Autodesk Fusion 360 part; units mm, degrees
note: some values were not read from the file. Set by a fixed rule: which sketch regions a step uses.
(part 9 of 20)
  spline S48 degree 5 poles (20.3781, 23.3609) (20.3757, 23.3596) (20.371, 23.3571) (20.3639, 23.3532) (20.3544, 23.348) (20.3426, 23.3416) (20.3308, 23.3351) (20.319, 23.3287) (20.3073, 23.3222) (20.2957, 23.3158) (20.284, 23.3094) (20.2724, 23.3029) (20.2609, 23.2965) (20.2493, 23.29) (20.2379, 23.2836) (20.2264, 23.2771) (20.215, 23.2707) (20.2036, 23.2643) (20.1922, 23.2578) (20.1809, 23.2514) (20.1697, 23.245) (20.1584, 23.2385) (20.1472, 23.2321) (20.136, 23.2257) (20.1249, 23.2193) (20.1138, 23.2128) (20.1028, 23.2064) (20.0917, 23.2) (20.0808, 23.1936) (20.0698, 23.1872) (20.0589, 23.1807) (20.048, 23.1743) (20.0372, 23.1679) (20.0264, 23.1615) (20.0156, 23.1551) (20.0049, 23.1487) (19.9942, 23.1423) (19.9836, 23.136) (19.973, 23.1296) (19.9624, 23.1232) (19.9518, 23.1168) (19.9413, 23.1104) (19.9309, 23.1041) (19.9205, 23.0977) (19.9101, 23.0914) (19.8997, 23.085) (19.8894, 23.0786) (19.8791, 23.0723) (19.8689, 23.066) (19.8587, 23.0596) (19.8486, 23.0533) (19.8384, 23.047) (19.8284, 23.0406) (19.8183, 23.0343) (19.8083, 23.028) (19.7984, 23.0217) (19.7884, 23.0154) (19.7785, 23.0091) (19.7687, 23.0029) (19.7589, 22.9966) (19.7491, 22.9903) (19.7394, 22.984) (19.7297, 22.9778) (19.72, 22.9715) (19.7104, 22.9653) (19.7009, 22.9591) (19.6913, 22.9528) (19.6818, 22.9466) (19.6724, 22.9404) (19.663, 22.9342) (19.6536, 22.928) (19.6443, 22.9218) (19.635, 22.9156) (19.6257, 22.9095) (19.6165, 22.9033) (19.6073, 22.8971) (19.5982, 22.891) (19.5891, 22.8849) (19.5801, 22.8787) (19.5711, 22.8726) (19.5621, 22.8665) (19.5532, 22.8604) (19.5443, 22.8543) (19.5354, 22.8483) (19.5266, 22.8422) (19.5179, 22.8361) (19.5091, 22.8301) (19.5005, 22.8241) (19.4918, 22.818) (19.4832, 22.812) (19.4747, 22.806) (19.4662, 22.8) (19.4577, 22.7941) (19.4493, 22.7881) (19.4409, 22.7822) (19.4325, 22.7762) (19.4242, 22.7703) (19.416, 22.7644) (19.4078, 22.7585) (19.3996, 22.7526) (19.3914, 22.7467) (19.3834, 22.7408) (19.3753, 22.735) (19.3673, 22.7292) (19.3593, 22.7233) (19.3514, 22.7175) (19.3436, 22.7118) (19.3357, 22.706) (19.3279, 22.7002) (19.3202, 22.6945) (19.3125, 22.6887) (19.3048, 22.683) (19.2972, 22.6773) (19.2897, 22.6716) (19.2821, 22.666) (19.2747, 22.6603) (19.2672, 22.6547) (19.2598, 22.6491) (19.2525, 22.6435) (19.2452, 22.6379) (19.2379, 22.6323) (19.2307, 22.6268) (19.2236, 22.6212) (19.2165, 22.6157) (19.2094, 22.6102) (19.2024, 22.6048) (19.1954, 22.5993) (19.1884, 22.5939) (19.1815, 22.5884) (19.1747, 22.583) (19.1679, 22.5777) (19.1611, 22.5723) (19.1544, 22.567) (19.1478, 22.5617) (19.1412, 22.5564) (19.1346, 22.5511) (19.1281, 22.5458) (19.1216, 22.5406) (19.1152, 22.5354) (19.1088, 22.5302) (19.1025, 22.525) (19.0962, 22.5199) (19.09, 22.5148) (19.0838, 22.5097) (19.0776, 22.5046) (19.0715, 22.4996) (19.0655, 22.4945) (19.0595, 22.4895) (19.0536, 22.4846) (19.0477, 22.4796) (19.0418, 22.4747) (19.036, 22.4698) (19.0303, 22.4649) (19.0246, 22.4601) (19.0189, 22.4553) (19.0133, 22.4505) (19.0077, 22.4457) (19.0022, 22.441) (18.9968, 22.4363) (18.9914, 22.4316) (18.986, 22.427) (18.9807, 22.4223) (18.9755, 22.4177) (18.9703, 22.4132) (18.9651, 22.4087) (18.96, 22.4042) (18.955, 22.3997) (18.95, 22.3953) (18.9451, 22.3909) (18.9402, 22.3865) (18.9353, 22.3821) (18.9306, 22.3778) (18.9258, 22.3736) (18.9211, 22.3693) (18.9165, 22.3651) (18.9119, 22.3609) (18.9074, 22.3568) (18.903, 22.3527) (18.8986, 22.3486) (18.8942, 22.3446) (18.8899, 22.3406) (18.8856, 22.3367) (18.8814, 22.3328) (18.8773, 22.3289) (18.8732, 22.325) (18.8692, 22.3212) (18.8652, 22.3175) (18.8613, 22.3138) (18.8574, 22.3101) (18.8536, 22.3065) (18.8499, 22.3029) (18.8462, 22.2993) (18.8426, 22.2958) (18.839, 22.2923) (18.8355, 22.2889) (18.832, 22.2855) (18.8286, 22.2822) (18.8252, 22.2789) (18.822, 22.2757) (18.8187, 22.2725) (18.8156, 22.2693) (18.8124, 22.2662) (18.8094, 22.2632) (18.8064, 22.2602) (18.8035, 22.2572) (18.8006, 22.2543) (18.7978, 22.2515) (18.7951, 22.2487) (18.7924, 22.2459) (18.7897, 22.2433) (18.7872, 22.2406) (18.7847, 22.238) (18.7823, 22.2355) (18.7799, 22.2331) (18.7776, 22.2307) (18.7753, 22.2283) (18.7732, 22.226) (18.771, 22.2238) (18.769, 22.2216) (18.767, 22.2195) (18.7651, 22.2175) (18.7632, 22.2155) (18.7615, 22.2136) (18.7597, 22.2117) (18.7581, 22.2099) (18.7565, 22.2082) (18.755, 22.2066) (18.7536, 22.205) (18.7522, 22.2035) (18.7509, 22.202) (18.7497, 22.2007) (18.7485, 22.1994) (18.7474, 22.1982) (18.7464, 22.197) (18.7455, 22.196) (18.7446, 22.195) (18.7438, 22.1941) (18.7431, 22.1933) (18.7424, 22.1925) (18.7419, 22.1919) (18.7414, 22.1913) (18.741, 22.1909) (18.7408, 22.1907) (18.7407, 22.1905) (18.7406, 22.1904) knots -1 -1 -1 -1 -1 -1 -0.99583333 -0.99166667 -0.9875 -0.98333333 -0.97916667 -0.975 -0.97083333 -0.96666667 -0.9625 -0.95833333 -0.95416667 -0.95 -0.94583333 -0.94166667 -0.9375 -0.93333333 -0.92916667 -0.925 -0.92083333 -0.91666667 -0.9125 -0.90833333 -0.90416667 -0.9 -0.89583333 -0.89166667 -0.8875 -0.88333333 -0.87916667 -0.875 -0.87083333 -0.86666667 -0.8625 -0.85833333 -0.85416667 -0.85 -0.84583333 -0.84166667 -0.8375 -0.83333333 -0.82916667 -0.825 -0.82083333 -0.81666667 -0.8125 -0.80833333 -0.80416667 -0.8 -0.79583333 -0.79166667 -0.7875 -0.78333333 -0.77916667 -0.775 -0.77083333 -0.76666667 -0.7625 -0.75833333 -0.75416667 -0.75 -0.74583333 -0.74166667 -0.7375 -0.73333333 -0.72916667 -0.725 -0.72083333 -0.71666667 -0.7125 -0.70833333 -0.70416667 -0.7 -0.69583333 -0.69166667 -0.6875 -0.68333333 -0.67916667 -0.675 -0.67083333 -0.66666667 -0.6625 -0.65833333 -0.65416667 -0.65 -0.64583333 -0.64166667 -0.6375 -0.63333333 -0.62916667 -0.625 -0.62083333 -0.61666667 -0.6125 -0.60833333 -0.60416667 -0.6 -0.59583333 -0.59166667 -0.5875 -0.58333333 -0.57916667 -0.575 -0.57083333 -0.56666667 -0.5625 -0.55833333 -0.55416667 -0.55 -0.54583333 -0.54166667 -0.5375 -0.53333333 -0.52916667 -0.525 -0.52083333 -0.51666667 -0.5125 -0.50833333 -0.50416667 -0.5 -0.49583333 -0.49166667 -0.4875 -0.48333333 -0.47916667 -0.475 -0.47083333 -0.46666667 -0.4625 -0.45833333 -0.45416667 -0.45 -0.44583333 -0.44166667 -0.4375 -0.43333333 -0.42916667 -0.425 -0.42083333 -0.41666667 -0.4125 -0.40833333 -0.40416667 -0.4 -0.39583333 -0.39166667 -0.3875 -0.38333333 -0.37916667 -0.375 -0.37083333 -0.36666667 -0.3625 -0.35833333 -0.35416667 -0.35 -0.34583333 -0.34166667 -0.3375 -0.33333333 -0.32916667 -0.325 -0.32083333 -0.31666667 -0.3125 -0.30833333 -0.30416667 -0.3 -0.29583333 -0.29166667 -0.2875 -0.28333333 -0.27916667 -0.275 -0.27083333 -0.26666667 -0.2625 -0.25833333 -0.25416667 -0.25 -0.24583333 -0.24166667 -0.2375 -0.23333333 -0.22916667 -0.225 -0.22083333 -0.21666667 -0.2125 -0.20833333 -0.20416667 -0.2 -0.19583333 -0.19166667 -0.1875 -0.18333333 -0.17916667 -0.175 -0.17083333 -0.16666667 -0.1625 -0.15833333 -0.15416667 -0.15 -0.14583333 -0.14166667 -0.1375 -0.13333333 -0.12916667 -0.125 -0.12083333 -0.11666667 -0.1125 -0.10833333 -0.10416667 -0.1 -0.09583333 -0.09166667 -0.0875 -0.08333333 -0.07916667 -0.075 -0.07083333 -0.06666667 -0.0625 -0.05833333 -0.05416667 -0.05 -0.04583333 -0.04166667 -0.0375 -0.03333333 -0.02916667 -0.025 -0.02083333 -0.01666667 -0.0125 -0.00833333 -0.00416667 0 0 0 0 0 0
  line L102 (27.8937, -8.0945) -> (27.6109, -8.0125)
  spline S49 degree 5 poles (30.8773, -2.755) (30.8749, -2.7539) (30.87, -2.7515) (30.8627, -2.748) (30.853, -2.7434) (30.8408, -2.7376) (30.8287, -2.7319) (30.8165, -2.7262) (30.8044, -2.7205) (30.7924, -2.7149) (30.7803, -2.7092) (30.7683, -2.7036) (30.7563, -2.6981) (30.7443, -2.6925) (30.7323, -2.687) (30.7204, -2.6815) (30.7085, -2.6761) (30.6966, -2.6707) (30.6847, -2.6653) (30.6728, -2.6599) (30.661, -2.6545) (30.6492, -2.6492) (30.6374, -2.6439) (30.6256, -2.6387) (30.6139, -2.6335) (30.6022, -2.6283) (30.5905, -2.6231) (30.5788, -2.6179) (30.5672, -2.6128) (30.5555, -2.6077) (30.5439, -2.6027) (30.5324, -2.5977) (30.5208, -2.5927) (30.5093, -2.5877) (30.4978, -2.5827) (30.4863, -2.5778) (30.4749, -2.5729) (30.4634, -2.5681) (30.452, -2.5632) (30.4407, -2.5584) (30.4293, -2.5537) (30.418, -2.5489) (30.4067, -2.5442) (30.3954, -2.5395) (30.3841, -2.5348) (30.3729, -2.5302) (30.3617, -2.5256) (30.3506, -2.521) (30.3394, -2.5165) (30.3283, -2.5119) (30.3172, -2.5074) (30.3061, -2.503) (30.2951, -2.4985) (30.2841, -2.4941) (30.2731, -2.4897) (30.2621, -2.4854) (30.2512, -2.481) (30.2403, -2.4767) (30.2294, -2.4725) (30.2186, -2.4682) (30.2078, -2.464) (30.197, -2.4598) (30.1862, -2.4557) (30.1755, -2.4515) (30.1648, -2.4474) (30.1541, -2.4433) (30.1435, -2.4393) (30.1329, -2.4353) (30.1223, -2.4313) (30.1118, -2.4273) (30.1012, -2.4234) (30.0907, -2.4194) (30.0803, -2.4156) (30.0699, -2.4117) (30.0595, -2.4079) (30.0491, -2.4041) (30.0388, -2.4003) (30.0284, -2.3965) (30.0182, -2.3928) (30.0079, -2.3891) (29.9977, -2.3855) (29.9875, -2.3818) (29.9774, -2.3782) (29.9673, -2.3746) (29.9572, -2.3711) (29.9471, -2.3675) (29.9371, -2.364) (29.9271, -2.3606) (29.9172, -2.3571) (29.9073, -2.3537) (29.8974, -2.3503) (29.8875, -2.3469) (29.8777, -2.3436) (29.868, -2.3403) (29.8582, -2.337) (29.8485, -2.3337) (29.8388, -2.3305) (29.8292, -2.3273) (29.8196, -2.3241) (29.81, -2.321) (29.8005, -2.3178) (29.791, -2.3147) (29.7815, -2.3117) (29.7721, -2.3086) (29.7627, -2.3056) (29.7534, -2.3026) (29.7441, -2.2996) (29.7348, -2.2967) (29.7255, -2.2938) (29.7163, -2.2909) (29.7072, -2.288) (29.6981, -2.2852) (29.689, -2.2824) (29.6799, -2.2796) (29.6709, -2.2769) (29.6619, -2.2741) (29.653, -2.2714) (29.6441, -2.2688) (29.6353, -2.2661) (29.6265, -2.2635) (29.6177, -2.2609) (29.609, -2.2583) (29.6003, -2.2558) (29.5917, -2.2533) (29.583, -2.2508) (29.5745, -2.2483) (29.566, -2.2458) (29.5575, -2.2434) (29.5491, -2.241) (29.5407, -2.2387) (29.5323, -2.2363) (29.524, -2.234) (29.5158, -2.2317) (29.5075, -2.2295) (29.4994, -2.2272) (29.4912, -2.225) (29.4832, -2.2228) (29.4751, -2.2207) (29.4671, -2.2185) (29.4592, -2.2164) (29.4513, -2.2143) (29.4434, -2.2123) (29.4356, -2.2102) (29.4279, -2.2082) (29.4202, -2.2062) (29.4125, -2.2043) (29.4049, -2.2023) (29.3973, -2.2004) (29.3898, -2.1985) (29.3823, -2.1967) (29.3749, -2.1948) (29.3675, -2.193) (29.3602, -2.1912) (29.3529, -2.1895) (29.3457, -2.1877) (29.3386, -2.186) (29.3314, -2.1843) (29.3244, -2.1827) (29.3174, -2.181) (29.3104, -2.1794) (29.3035, -2.1778) (29.2967, -2.1762) (29.2899, -2.1747) (29.2831, -2.1731) (29.2764, -2.1716) (29.2698, -2.1702) (29.2632, -2.1687) (29.2567, -2.1673) (29.2502, -2.1659) (29.2438, -2.1645) (29.2374, -2.1631) (29.2311, -2.1618) (29.2249, -2.1605) (29.2187, -2.1592) (29.2126, -2.1579) (29.2065, -2.1567) (29.2005, -2.1554) (29.1946, -2.1542) (29.1887, -2.153) (29.1829, -2.1519) (29.1771, -2.1507) (29.1714, -2.1496) (29.1658, -2.1485) (29.1602, -2.1475) (29.1547, -2.1464) (29.1493, -2.1454) (29.1439, -2.1444) (29.1386, -2.1434) (29.1334, -2.1424) (29.1282, -2.1415) (29.1231, -2.1406) (29.118, -2.1397) (29.1131, -2.1388) (29.1081, -2.138) (29.1033, -2.1371) (29.0985, -2.1363) (29.0938, -2.1355) (29.0892, -2.1347) (29.0847, -2.134) (29.0802, -2.1332) (29.0758, -2.1325) (29.0714, -2.1318) (29.0672, -2.1312) (29.063, -2.1305) (29.0589, -2.1299) (29.0549, -2.1292) (29.0509, -2.1286) (29.047, -2.1281) (29.0432, -2.1275) (29.0395, -2.127) (29.0359, -2.1264) (29.0323, -2.1259) (29.0289, -2.1254) (29.0255, -2.125) (29.0222, -2.1245) (29.0189, -2.1241) (29.0158, -2.1237) (29.0128, -2.1233) (29.0098, -2.1229) (29.0069, -2.1225) (29.0041, -2.1222) (29.0015, -2.1219) (28.9989, -2.1215) (28.9963, -2.1212) (28.9939, -2.121) (28.9916, -2.1207) (28.9894, -2.1204) (28.9873, -2.1202) (28.9852, -2.12) (28.9833, -2.1198) (28.9815, -2.1196) (28.9798, -2.1194) (28.9781, -2.1192) (28.9766, -2.1191) (28.9752, -2.1189) (28.9739, -2.1188) (28.9727, -2.1187) (28.9716, -2.1186) (28.9706, -2.1185) (28.9698, -2.1184) (28.969, -2.1184) (28.9685, -2.1183) (28.9682, -2.1183) (28.968, -2.1183) (28.9679, -2.1183) knots -1 -1 -1 -1 -1 -1 -0.99583333 -0.99166667 -0.9875 -0.98333333 -0.97916667 -0.975 -0.97083333 -0.96666667 -0.9625 -0.95833333 -0.95416667 -0.95 -0.94583333 -0.94166667 -0.9375 -0.93333333 -0.92916667 -0.925 -0.92083333 -0.91666667 -0.9125 -0.90833333 -0.90416667 -0.9 -0.89583333 -0.89166667 -0.8875 -0.88333333 -0.87916667 -0.875 -0.87083333 -0.86666667 -0.8625 -0.85833333 -0.85416667 -0.85 -0.84583333 -0.84166667 -0.8375 -0.83333333 -0.82916667 -0.825 -0.82083333 -0.81666667 -0.8125 -0.80833333 -0.80416667 -0.8 -0.79583333 -0.79166667 -0.7875 -0.78333333 -0.77916667 -0.775 -0.77083333 -0.76666667 -0.7625 -0.75833333 -0.75416667 -0.75 -0.74583333 -0.74166667 -0.7375 -0.73333333 -0.72916667 -0.725 -0.72083333 -0.71666667 -0.7125 -0.70833333 -0.70416667 -0.7 -0.69583333 -0.69166667 -0.6875 -0.68333333 -0.67916667 -0.675 -0.67083333 -0.66666667 -0.6625 -0.65833333 -0.65416667 -0.65 -0.64583333 -0.64166667 -0.6375 -0.63333333 -0.62916667 -0.625 -0.62083333 -0.61666667 -0.6125 -0.60833333 -0.60416667 -0.6 -0.59583333 -0.59166667 -0.5875 -0.58333333 -0.57916667 -0.575 -0.57083333 -0.56666667 -0.5625 -0.55833333 -0.55416667 -0.55 -0.54583333 -0.54166667 -0.5375 -0.53333333 -0.52916667 -0.525 -0.52083333 -0.51666667 -0.5125 -0.50833333 -0.50416667 -0.5 -0.49583333 -0.49166667 -0.4875 -0.48333333 -0.47916667 -0.475 -0.47083333 -0.46666667 -0.4625 -0.45833333 -0.45416667 -0.45 -0.44583333 -0.44166667 -0.4375 -0.43333333 -0.42916667 -0.425 -0.42083333 -0.41666667 -0.4125 -0.40833333 -0.40416667 -0.4 -0.39583333 -0.39166667 -0.3875 -0.38333333 -0.37916667 -0.375 -0.37083333 -0.36666667 -0.3625 -0.35833333 -0.35416667 -0.35 -0.34583333 -0.34166667 -0.3375 -0.33333333 -0.32916667 -0.325 -0.32083333 -0.31666667 -0.3125 -0.30833333 -0.30416667 -0.3 -0.29583333 -0.29166667 -0.2875 -0.28333333 -0.27916667 -0.275 -0.27083333 -0.26666667 -0.2625 -0.25833333 -0.25416667 -0.25 -0.24583333 -0.24166667 -0.2375 -0.23333333 -0.22916667 -0.225 -0.22083333 -0.21666667 -0.2125 -0.20833333 -0.20416667 -0.2 -0.19583333 -0.19166667 -0.1875 -0.18333333 -0.17916667 -0.175 -0.17083333 -0.16666667 -0.1625 -0.15833333 -0.15416667 -0.15 -0.14583333 -0.14166667 -0.1375 -0.13333333 -0.12916667 -0.125 -0.12083333 -0.11666667 -0.1125 -0.10833333 -0.10416667 -0.1 -0.09583333 -0.09166667 -0.0875 -0.08333333 -0.07916667 -0.075 -0.07083333 -0.06666667 -0.0625 -0.05833333 -0.05416667 -0.05 -0.04583333 -0.04166667 -0.0375 -0.03333333 -0.02916667 -0.025 -0.02083333 -0.01666667 -0.0125 -0.00833333 -0.00416667 0 0 0 0 0 0
  spline S50 degree 5 poles (-26.5997, -15.9204) (-26.597, -15.9199) (-26.5917, -15.9189) (-26.5837, -15.9174) (-26.5731, -15.9154) (-26.5599, -15.913) (-26.5467, -15.9105) (-26.5335, -15.908) (-26.5204, -15.9055) (-26.5073, -15.9029) (-26.4943, -15.9004) (-26.4812, -15.8979) (-26.4682, -15.8953) (-26.4553, -15.8927) (-26.4424, -15.8902) (-26.4295, -15.8876) (-26.4166, -15.885) (-26.4038, -15.8824) (-26.391, -15.8798) (-26.3783, -15.8771) (-26.3656, -15.8745) (-26.3529, -15.8719) (-26.3403, -15.8692) (-26.3276, -15.8666) (-26.3151, -15.8639) (-26.3025, -15.8612) (-26.29, -15.8585) (-26.2776, -15.8558) (-26.2651, -15.8531) (-26.2528, -15.8504) (-26.2404, -15.8477) (-26.2281, -15.8449) (-26.2158, -15.8422) (-26.2035, -15.8394) (-26.1913, -15.8367) (-26.1792, -15.8339) (-26.167, -15.8311) (-26.1549, -15.8283) (-26.1428, -15.8255) (-26.1308, -15.8227) (-26.1188, -15.8199) (-26.1069, -15.8171) (-26.095, -15.8143) (-26.0831, -15.8115) (-26.0712, -15.8086) (-26.0594, -15.8058) (-26.0477, -15.8029) (-26.0359, -15.8001) (-26.0242, -15.7972) (-26.0126, -15.7943) (-26.001, -15.7914) (-25.9894, -15.7886) (-25.9778, -15.7857) (-25.9663, -15.7828) (-25.9549, -15.7798) (-25.9435, -15.7769) (-25.9321, -15.774) (-25.9207, -15.7711) (-25.9094, -15.7682) (-25.8982, -15.7652) (-25.8869, -15.7623) (-25.8757, -15.7593) (-25.8646, -15.7564) (-25.8535, -15.7534) (-25.8424, -15.7504) (-25.8314, -15.7475) (-25.8204, -15.7445) (-25.8094, -15.7415) (-25.7985, -15.7385) (-25.7877, -15.7355) (-25.7768, -15.7325) (-25.766, -15.7295) (-25.7553, -15.7265) (-25.7446, -15.7235) (-25.7339, -15.7205) (-25.7233, -15.7175) (-25.7127, -15.7145) (-25.7022, -15.7114) (-25.6917, -15.7084) (-25.6812, -15.7054) (-25.6708, -15.7023) (-25.6604, -15.6993) (-25.6501, -15.6963) (-25.6398, -15.6932) (-25.6296, -15.6902) (-25.6194, -15.6871) (-25.6092, -15.6841) (-25.5991, -15.681) (-25.589, -15.6779) (-25.579, -15.6749) (-25.569, -15.6718) (-25.559, -15.6688) (-25.5491, -15.6657) (-25.5393, -15.6626) (-25.5294, -15.6596) (-25.5197, -15.6565) (-25.5099, -15.6534) (-25.5003, -15.6503) (-25.4906, -15.6473) (-25.481, -15.6442) (-25.4715, -15.6411) (-25.462, -15.638) (-25.4525, -15.635) (-25.4431, -15.6319) (-25.4337, -15.6288) (-25.4244, -15.6257) (-25.4151, -15.6227) (-25.4059, -15.6196) (-25.3967, -15.6165) (-25.3876, -15.6134) (-25.3785, -15.6104) (-25.3694, -15.6073) (-25.3604, -15.6042) (-25.3515, -15.6012) (-25.3426, -15.5981) (-25.3337, -15.595) (-25.3249, -15.592) (-25.3161, -15.5889) (-25.3074, -15.5859) (-25.2988, -15.5828) (-25.2901, -15.5798) (-25.2816, -15.5767) (-25.2731, -15.5737) (-25.2646, -15.5706) (-25.2562, -15.5676) (-25.2478, -15.5645) (-25.2394, -15.5615) (-25.2312, -15.5585) (-25.2229, -15.5555) (-25.2148, -15.5524) (-25.2066, -15.5494) (-25.1986, -15.5464) (-25.1905, -15.5434) (-25.1826, -15.5404) (-25.1746, -15.5374) (-25.1668, -15.5344) (-25.1589, -15.5315) (-25.1512, -15.5285) (-25.1434, -15.5255) (-25.1358, -15.5226) (-25.1282, -15.5196) (-25.1206, -15.5166) (-25.1131, -15.5137) (-25.1056, -15.5108) (-25.0982, -15.5078) (-25.0909, -15.5049) (-25.0836, -15.502) (-25.0763, -15.4991) (-25.0691, -15.4962) (-25.062, -15.4933) (-25.0549, -15.4905) (-25.0479, -15.4876) (-25.0409, -15.4848) (-25.034, -15.4819) (-25.0271, -15.4791) (-25.0203, -15.4762) (-25.0136, -15.4734) (-25.0069, -15.4706) (-25.0002, -15.4678) (-24.9936, -15.4651) (-24.9871, -15.4623) (-24.9806, -15.4595) (-24.9742, -15.4568) (-24.9679, -15.4541) (-24.9616, -15.4514) (-24.9553, -15.4486) (-24.9492, -15.446) (-24.943, -15.4433) (-24.937, -15.4406) (-24.931, -15.438) (-24.925, -15.4353) (-24.9192, -15.4327) (-24.9133, -15.4301) (-24.9076, -15.4275) (-24.9019, -15.425) (-24.8962, -15.4224) (-24.8907, -15.4199) (-24.8852, -15.4174) (-24.8797, -15.4149) (-24.8743, -15.4124) (-24.869, -15.4099) (-24.8637, -15.4075) (-24.8585, -15.405) (-24.8534, -15.4026) (-24.8483, -15.4002) (-24.8433, -15.3979) (-24.8384, -15.3955) (-24.8335, -15.3932) (-24.8287, -15.3909) (-24.8239, -15.3886) (-24.8193, -15.3863) (-24.8147, -15.3841) (-24.8101, -15.3819) (-24.8056, -15.3797) (-24.8012, -15.3775) (-24.7969, -15.3754) (-24.7926, -15.3733) (-24.7884, -15.3712) (-24.7843, -15.3691) (-24.7802, -15.3671) (-24.7763, -15.3651) (-24.7723, -15.3631) (-24.7685, -15.3611) (-24.7647, -15.3592) (-24.761, -15.3573) (-24.7574, -15.3554) (-24.7539, -15.3536) (-24.7504, -15.3518) (-24.747, -15.35) (-24.7437, -15.3482) (-24.7404, -15.3465) (-24.7372, -15.3449) (-24.7341, -15.3432) (-24.7311, -15.3416) (-24.7282, -15.34) (-24.7253, -15.3385) (-24.7225, -15.337) (-24.7198, -15.3355) (-24.7172, -15.3341) (-24.7147, -15.3327) (-24.7122, -15.3313) (-24.7099, -15.33) (-24.7076, -15.3287) (-24.7054, -15.3275) (-24.7033, -15.3263) (-24.7012, -15.3252) (-24.6993, -15.3241) (-24.6974, -15.323) (-24.6956, -15.322) (-24.694, -15.321) (-24.6924, -15.3201) (-24.6909, -15.3193) (-24.6895, -15.3184) (-24.6881, -15.3177) (-24.6869, -15.3169) (-24.6858, -15.3163) (-24.6848, -15.3157) (-24.6838, -15.3151) (-24.683, -15.3146) (-24.6822, -15.3142) (-24.6816, -15.3138) (-24.6812, -15.3135) (-24.6809, -15.3133) (-24.6807, -15.3132) (-24.6806, -15.3132) knots -1 -1 -1 -1 -1 -1 -0.99583333 -0.99166667 -0.9875 -0.98333333 -0.97916667 -0.975 -0.97083333 -0.96666667 -0.9625 -0.95833333 -0.95416667 -0.95 -0.94583333 -0.94166667 -0.9375 -0.93333333 -0.92916667 -0.925 -0.92083333 -0.91666667 -0.9125 -0.90833333 -0.90416667 -0.9 -0.89583333 -0.89166667 -0.8875 -0.88333333 -0.87916667 -0.875 -0.87083333 -0.86666667 -0.8625 -0.85833333 -0.85416667 -0.85 -0.84583333 -0.84166667 -0.8375 -0.83333333 -0.82916667 -0.825 -0.82083333 -0.81666667 -0.8125 -0.80833333 -0.80416667 -0.8 -0.79583333 -0.79166667 -0.7875 -0.78333333 -0.77916667 -0.775 -0.77083333 -0.76666667 -0.7625 -0.75833333 -0.75416667 -0.75 -0.74583333 -0.74166667 -0.7375 -0.73333333 -0.72916667 -0.725 -0.72083333 -0.71666667 -0.7125 -0.70833333 -0.70416667 -0.7 -0.69583333 -0.69166667 -0.6875 -0.68333333 -0.67916667 -0.675 -0.67083333 -0.66666667 -0.6625 -0.65833333 -0.65416667 -0.65 -0.64583333 -0.64166667 -0.6375 -0.63333333 -0.62916667 -0.625 -0.62083333 -0.61666667 -0.6125 -0.60833333 -0.60416667 -0.6 -0.59583333 -0.59166667 -0.5875 -0.58333333 -0.57916667 -0.575 -0.57083333 -0.56666667 -0.5625 -0.55833333 -0.55416667 -0.55 -0.54583333 -0.54166667 -0.5375 -0.53333333 -0.52916667 -0.525 -0.52083333 -0.51666667 -0.5125 -0.50833333 -0.50416667 -0.5 -0.49583333 -0.49166667 -0.4875 -0.48333333 -0.47916667 -0.475 -0.47083333 -0.46666667 -0.4625 -0.45833333 -0.45416667 -0.45 -0.44583333 -0.44166667 -0.4375 -0.43333333 -0.42916667 -0.425 -0.42083333 -0.41666667 -0.4125 -0.40833333 -0.40416667 -0.4 -0.39583333 -0.39166667 -0.3875 -0.38333333 -0.37916667 -0.375 -0.37083333 -0.36666667 -0.3625 -0.35833333 -0.35416667 -0.35 -0.34583333 -0.34166667 -0.3375 -0.33333333 -0.32916667 -0.325 -0.32083333 -0.31666667 -0.3125 -0.30833333 -0.30416667 -0.3 -0.29583333 -0.29166667 -0.2875 -0.28333333 -0.27916667 -0.275 -0.27083333 -0.26666667 -0.2625 -0.25833333 -0.25416667 -0.25 -0.24583333 -0.24166667 -0.2375 -0.23333333 -0.22916667 -0.225 -0.22083333 -0.21666667 -0.2125 -0.20833333 -0.20416667 -0.2 -0.19583333 -0.19166667 -0.1875 -0.18333333 -0.17916667 -0.175 -0.17083333 -0.16666667 -0.1625 -0.15833333 -0.15416667 -0.15 -0.14583333 -0.14166667 -0.1375 -0.13333333 -0.12916667 -0.125 -0.12083333 -0.11666667 -0.1125 -0.10833333 -0.10416667 -0.1 -0.09583333 -0.09166667 -0.0875 -0.08333333 -0.07916667 -0.075 -0.07083333 -0.06666667 -0.0625 -0.05833333 -0.05416667 -0.05 -0.04583333 -0.04166667 -0.0375 -0.03333333 -0.02916667 -0.025 -0.02083333 -0.01666667 -0.0125 -0.00833333 -0.00416667 0 0 0 0 0 0
  line L103 (26.1453, -12.6491) -> (26.1461, -12.6495)
  line L104 (27.0473, -9.7471) -> (27.3243, -9.8469)
  arc A53 (-24.4297, -15.1575) -> (-23.7836, -16.1526) centre (0, 0) ccw
  arc A54 (25.3417, -13.578) -> (25.8803, -12.5209) centre (0, 0) ccw
  line L105 (25.8803, -12.5209) -> (26.1453, -12.6491)
  spline S51 degree 5 poles (-28.1181, -13.0527) (-28.1154, -13.0525) (-28.11, -13.0521) (-28.1019, -13.0515) (-28.0911, -13.0506) (-28.0777, -13.0495) (-28.0644, -13.0484) (-28.051, -13.0473) (-28.0377, -13.0462) (-28.0244, -13.0451) (-28.0112, -13.0439) (-27.9979, -13.0427) (-27.9848, -13.0415) (-27.9716, -13.0404) (-27.9585, -13.0391) (-27.9454, -13.0379) (-27.9323, -13.0367) (-27.9193, -13.0354) (-27.9063, -13.0342) (-27.8934, -13.0329) (-27.8805, -13.0316) (-27.8676, -13.0303) (-27.8547, -13.029) (-27.8419, -13.0276) (-27.8291, -13.0263) (-27.8164, -13.0249) (-27.8037, -13.0236) (-27.791, -13.0222) (-27.7784, -13.0208) (-27.7658, -13.0194) (-27.7532, -13.018) (-27.7406, -13.0165) (-27.7281, -13.0151) (-27.7157, -13.0136) (-27.7032, -13.0122) (-27.6908, -13.0107) (-27.6785, -13.0092) (-27.6661, -13.0077) (-27.6539, -13.0062) (-27.6416, -13.0047) (-27.6294, -13.0031) (-27.6172, -13.0016) (-27.605, -13) (-27.5929, -12.9984) (-27.5809, -12.9968) (-27.5688, -12.9952) (-27.5568, -12.9936) (-27.5449, -12.992) (-27.5329, -12.9904) (-27.521, -12.9887) (-27.5092, -12.9871) (-27.4974, -12.9854) (-27.4856, -12.9838) (-27.4738, -12.9821) (-27.4621, -12.9804) (-27.4505, -12.9787) (-27.4388, -12.977) (-27.4273, -12.9752) (-27.4157, -12.9735) (-27.4042, -12.9718) (-27.3927, -12.97) (-27.3813, -12.9682) (-27.3699, -12.9665) (-27.3585, -12.9647) (-27.3472, -12.9629) (-27.3359, -12.9611) (-27.3247, -12.9593) (-27.3135, -12.9574) (-27.3023, -12.9556) (-27.2912, -12.9538) (-27.2801, -12.9519) (-27.2691, -12.9501) (-27.2581, -12.9482) (-27.2471, -12.9463) (-27.2362, -12.9445) (-27.2253, -12.9426) (-27.2145, -12.9407) (-27.2037, -12.9388) (-27.1929, -12.9368) (-27.1822, -12.9349) (-27.1715, -12.933) (-27.1609, -12.9311) (-27.1503, -12.9291) (-27.1397, -12.9272) (-27.1292, -12.9252) (-27.1188, -12.9232) (-27.1083, -12.9213) (-27.0979, -12.9193) (-27.0876, -12.9173) (-27.0773, -12.9153) (-27.0671, -12.9133) (-27.0568, -12.9113) (-27.0467, -12.9093) (-27.0365, -12.9072) (-27.0265, -12.9052) (-27.0164, -12.9032) (-27.0064, -12.9011) (-26.9965, -12.8991) (-26.9866, -12.8971) (-26.9767, -12.895) (-26.9669, -12.8929) (-26.9571, -12.8909) (-26.9474, -12.8888) (-26.9377, -12.8867) (-26.9281, -12.8847) (-26.9185, -12.8826) (-26.9089, -12.8805) (-26.8994, -12.8784) (-26.89, -12.8763) (-26.8806, -12.8742) (-26.8712, -12.8721) (-26.8619, -12.87) (-26.8526, -12.8679) (-26.8434, -12.8658) (-26.8342, -12.8636) (-26.8251, -12.8615) (-26.816, -12.8594) (-26.8069, -12.8573) (-26.798, -12.8551) (-26.789, -12.853) (-26.7801, -12.8509) (-26.7713, -12.8487) (-26.7625, -12.8466) (-26.7537, -12.8445) (-26.7451, -12.8423) (-26.7364, -12.8402) (-26.7278, -12.838) (-26.7193, -12.8359) (-26.7108, -12.8337) (-26.7023, -12.8316) (-26.6939, -12.8294) (-26.6856, -12.8273) (-26.6773, -12.8251) (-26.669, -12.823) (-26.6608, -12.8208) (-26.6527, -12.8187) (-26.6446, -12.8166) (-26.6365, -12.8144) (-26.6286, -12.8123) (-26.6206, -12.8101) (-26.6127, -12.808) (-26.6049, -12.8058) (-26.5971, -12.8037) (-26.5894, -12.8016) (-26.5817, -12.7994) (-26.5741, -12.7973) (-26.5665, -12.7952) (-26.559, -12.793) (-26.5516, -12.7909) (-26.5442, -12.7888) (-26.5368, -12.7867) (-26.5296, -12.7845) (-26.5223, -12.7824) (-26.5151, -12.7803) (-26.508, -12.7782) (-26.5009, -12.7761) (-26.4939, -12.774) (-26.487, -12.772) (-26.4801, -12.7699) (-26.4733, -12.7678) (-26.4665, -12.7657) (-26.4598, -12.7637) (-26.4531, -12.7616) (-26.4465, -12.7596) (-26.4399, -12.7575) (-26.4335, -12.7555) (-26.427, -12.7534) (-26.4207, -12.7514) (-26.4144, -12.7494) (-26.4081, -12.7474) (-26.4019, -12.7454) (-26.3958, -12.7434) (-26.3897, -12.7414) (-26.3837, -12.7395) (-26.3778, -12.7375) (-26.3719, -12.7356) (-26.3661, -12.7336) (-26.3604, -12.7317) (-26.3547, -12.7298) (-26.3491, -12.7279) (-26.3435, -12.726) (-26.338, -12.7241) (-26.3326, -12.7222) (-26.3273, -12.7204) (-26.322, -12.7185) (-26.3167, -12.7167) (-26.3116, -12.7149) (-26.3065, -12.7131) (-26.3015, -12.7113) (-26.2965, -12.7095) (-26.2916, -12.7077) (-26.2868, -12.706) (-26.282, -12.7043) (-26.2774, -12.7026) (-26.2728, -12.7009) (-26.2682, -12.6992) (-26.2638, -12.6975) (-26.2594, -12.6959) (-26.255, -12.6943) (-26.2508, -12.6927) (-26.2466, -12.6911) (-26.2425, -12.6895) (-26.2385, -12.688) (-26.2345, -12.6864) (-26.2307, -12.6849) (-26.2269, -12.6834) (-26.2231, -12.682) (-26.2195, -12.6806) (-26.2159, -12.6791) (-26.2124, -12.6778) (-26.209, -12.6764) (-26.2057, -12.675) (-26.2024, -12.6737) (-26.1993, -12.6724) (-26.1962, -12.6712) (-26.1932, -12.6699) (-26.1903, -12.6687) (-26.1874, -12.6676) (-26.1847, -12.6664) (-26.182, -12.6653) (-26.1794, -12.6642) (-26.1769, -12.6631) (-26.1745, -12.6621) (-26.1722, -12.6611) (-26.17, -12.6602) (-26.1678, -12.6592) (-26.1658, -12.6583) (-26.1638, -12.6575) (-26.1619, -12.6567) (-26.1602, -12.6559) (-26.1585, -12.6551) (-26.1569, -12.6544) (-26.1554, -12.6538) (-26.154, -12.6531) (-26.1527, -12.6526) (-26.1515, -12.652) (-26.1504, -12.6515) (-26.1495, -12.651) (-26.1486, -12.6506) (-26.1478, -12.6503) (-26.1471, -12.65) (-26.1467, -12.6497) (-26.1464, -12.6496) (-26.1462, -12.6495) (-26.1461, -12.6495) knots -1 -1 -1 -1 -1 -1 -0.99583333 -0.99166667 -0.9875 -0.98333333 -0.97916667 -0.975 -0.97083333 -0.96666667 -0.9625 -0.95833333 -0.95416667 -0.95 -0.94583333 -0.94166667 -0.9375 -0.93333333 -0.92916667 -0.925 -0.92083333 -0.91666667 -0.9125 -0.90833333 -0.90416667 -0.9 -0.89583333 -0.89166667 -0.8875 -0.88333333 -0.87916667 -0.875 -0.87083333 -0.86666667 -0.8625 -0.85833333 -0.85416667 -0.85 -0.84583333 -0.84166667 -0.8375 -0.83333333 -0.82916667 -0.825 -0.82083333 -0.81666667 -0.8125 -0.80833333 -0.80416667 -0.8 -0.79583333 -0.79166667 -0.7875 -0.78333333 -0.77916667 -0.775 -0.77083333 -0.76666667 -0.7625 -0.75833333 -0.75416667 -0.75 -0.74583333 -0.74166667 -0.7375 -0.73333333 -0.72916667 -0.725 -0.72083333 -0.71666667 -0.7125 -0.70833333 -0.70416667 -0.7 -0.69583333 -0.69166667 -0.6875 -0.68333333 -0.67916667 -0.675 -0.67083333 -0.66666667 -0.6625 -0.65833333 -0.65416667 -0.65 -0.64583333 -0.64166667 -0.6375 -0.63333333 -0.62916667 -0.625 -0.62083333 -0.61666667 -0.6125 -0.60833333 -0.60416667 -0.6 -0.59583333 -0.59166667 -0.5875 -0.58333333 -0.57916667 -0.575 -0.57083333 -0.56666667 -0.5625 -0.55833333 -0.55416667 -0.55 -0.54583333 -0.54166667 -0.5375 -0.53333333 -0.52916667 -0.525 -0.52083333 -0.51666667 -0.5125 -0.50833333 -0.50416667 -0.5 -0.49583333 -0.49166667 -0.4875 -0.48333333 -0.47916667 -0.475 -0.47083333 -0.46666667 -0.4625 -0.45833333 -0.45416667 -0.45 -0.44583333 -0.44166667 -0.4375 -0.43333333 -0.42916667 -0.425 -0.42083333 -0.41666667 -0.4125 -0.40833333 -0.40416667 -0.4 -0.39583333 -0.39166667 -0.3875 -0.38333333 -0.37916667 -0.375 -0.37083333 -0.36666667 -0.3625 -0.35833333 -0.35416667 -0.35 -0.34583333 -0.34166667 -0.3375 -0.33333333 -0.32916667 -0.325 -0.32083333 -0.31666667 -0.3125 -0.30833333 -0.30416667 -0.3 -0.29583333 -0.29166667 -0.2875 -0.28333333 -0.27916667 -0.275 -0.27083333 -0.26666667 -0.2625 -0.25833333 -0.25416667 -0.25 -0.24583333 -0.24166667 -0.2375 -0.23333333 -0.22916667 -0.225 -0.22083333 -0.21666667 -0.2125 -0.20833333 -0.20416667 -0.2 -0.19583333 -0.19166667 -0.1875 -0.18333333 -0.17916667 -0.175 -0.17083333 -0.16666667 -0.1625 -0.15833333 -0.15416667 -0.15 -0.14583333 -0.14166667 -0.1375 -0.13333333 -0.12916667 -0.125 -0.12083333 -0.11666667 -0.1125 -0.10833333 -0.10416667 -0.1 -0.09583333 -0.09166667 -0.0875 -0.08333333 -0.07916667 -0.075 -0.07083333 -0.06666667 -0.0625 -0.05833333 -0.05416667 -0.05 -0.04583333 -0.04166667 -0.0375 -0.03333333 -0.02916667 -0.025 -0.02083333 -0.01666667 -0.0125 -0.00833333 -0.00416667 0 0 0 0 0 0
  line L106 (26.8955, -10.9662) -> (26.8948, -10.9659)
  arc A55 (-27.0873, -15.0758) -> (-26.5997, -15.9204) centre (0, 0) ccw
  line L107 (-28.2047, -6.937) -> (-28.2039, -6.9368)
  line L108 (22.1898, -18.7401) -> (21.9649, -18.5501)
  line L109 (-27.6109, -8.0125) -> (-27.8937, -8.0945)
  spline S52 degree 5 poles (-28.5878, -5.1346) (-28.5879, -5.1347) (-28.5881, -5.1347) (-28.5884, -5.1348) (-28.5889, -5.1349) (-28.5896, -5.135) (-28.5905, -5.1352) (-28.5915, -5.1354) (-28.5925, -5.1356) (-28.5937, -5.1358) (-28.595, -5.1361) (-28.5964, -5.1363) (-28.5979, -5.1367) (-28.5995, -5.137) (-28.6012, -5.1374) (-28.603, -5.1377) (-28.6049, -5.1381) (-28.6069, -5.1386) (-28.6089, -5.139) (-28.6111, -5.1395) (-28.6134, -5.14) (-28.6158, -5.1406) (-28.6182, -5.1411) (-28.6208, -5.1417) (-28.6234, -5.1423) (-28.6262, -5.143) (-28.629, -5.1436) (-28.6319, -5.1443) (-28.6349, -5.145) (-28.6379, -5.1458) (-28.6411, -5.1465) (-28.6443, -5.1473) (-28.6477, -5.1481) (-28.6511, -5.149) (-28.6545, -5.1499) (-28.6581, -5.1508) (-28.6617, -5.1517) (-28.6655, -5.1527) (-28.6693, -5.1536) (-28.6731, -5.1546) (-28.6771, -5.1557) (-28.6811, -5.1567) (-28.6852, -5.1578) (-28.6893, -5.1589) (-28.6936, -5.1601) (-28.6979, -5.1613) (-28.7023, -5.1625) (-28.7067, -5.1637) (-28.7112, -5.1649) (-28.7158, -5.1662) (-28.7205, -5.1675) (-28.7252, -5.1689) (-28.73, -5.1702) (-28.7349, -5.1716) (-28.7398, -5.173) (-28.7448, -5.1745) (-28.7498, -5.176) (-28.7549, -5.1775) (-28.7601, -5.179) (-28.7654, -5.1806) (-28.7707, -5.1822) (-28.776, -5.1838) (-28.7815, -5.1854) (-28.7869, -5.1871) (-28.7925, -5.1888) (-28.7981, -5.1905) (-28.8038, -5.1923) (-28.8095, -5.1941) (-28.8153, -5.1959) (-28.8211, -5.1978) (-28.827, -5.1996) (-28.833, -5.2015) (-28.839, -5.2035) (-28.8451, -5.2054) (-28.8512, -5.2074) (-28.8573, -5.2094) (-28.8636, -5.2115) (-28.8699, -5.2136) (-28.8762, -5.2157) (-28.8826, -5.2178) (-28.889, -5.22) (-28.8955, -5.2222) (-28.9021, -5.2244) (-28.9087, -5.2266) (-28.9153, -5.2289) (-28.922, -5.2312) (-28.9288, -5.2336) (-28.9356, -5.2359) (-28.9424, -5.2383) (-28.9493, -5.2408) (-28.9563, -5.2432) (-28.9633, -5.2457) (-28.9703, -5.2482) (-28.9774, -5.2508) (-28.9846, -5.2533) (-28.9918, -5.2559) (-28.999, -5.2586) (-29.0063, -5.2612) (-29.0136, -5.2639) (-29.021, -5.2666) (-29.0284, -5.2694) (-29.0358, -5.2722) (-29.0433, -5.275) (-29.0509, -5.2778) (-29.0585, -5.2807) (-29.0661, -5.2836) (-29.0738, -5.2865) (-29.0815, -5.2895) (-29.0893, -5.2925) (-29.0971, -5.2955) (-29.105, -5.2986) (-29.1129, -5.3016) (-29.1208, -5.3047) (-29.1288, -5.3079) (-29.1368, -5.3111) (-29.1448, -5.3143) (-29.1529, -5.3175) (-29.1611, -5.3207) (-29.1692, -5.324) (-29.1775, -5.3273) (-29.1857, -5.3307) (-29.194, -5.3341) (-29.2023, -5.3375) (-29.2107, -5.3409) (-29.2191, -5.3444) (-29.2276, -5.3479) (-29.2361, -5.3514) (-29.2446, -5.355) (-29.2531, -5.3586) (-29.2617, -5.3622) (-29.2704, -5.3658) (-29.279, -5.3695) (-29.2878, -5.3732) (-29.2965, -5.377) (-29.3053, -5.3807) (-29.3141, -5.3846) (-29.3229, -5.3884) (-29.3318, -5.3922) (-29.3407, -5.3961) (-29.3497, -5.4001) (-29.3587, -5.404) (-29.3677, -5.408) (-29.3767, -5.412) (-29.3858, -5.4161) (-29.395, -5.4201) (-29.4041, -5.4242) (-29.4133, -5.4284) (-29.4225, -5.4325) (-29.4318, -5.4367) (-29.441, -5.441) (-29.4504, -5.4452) (-29.4597, -5.4495) (-29.4691, -5.4538) (-29.4785, -5.4582) (-29.4879, -5.4625) (-29.4974, -5.467) (-29.5069, -5.4714) (-29.5165, -5.4759) (-29.526, -5.4804) (-29.5356, -5.4849) (-29.5452, -5.4895) (-29.5549, -5.494) (-29.5646, -5.4987) (-29.5743, -5.5033) (-29.584, -5.508) (-29.5938, -5.5127) (-29.6036, -5.5175) (-29.6134, -5.5222) (-29.6233, -5.527) (-29.6332, -5.5319) (-29.6431, -5.5367) (-29.653, -5.5416) (-29.663, -5.5466) (-29.673, -5.5515) (-29.683, -5.5565) (-29.6931, -5.5615) (-29.7032, -5.5666) (-29.7133, -5.5717) (-29.7234, -5.5768) (-29.7336, -5.5819) (-29.7437, -5.5871) (-29.754, -5.5923) (-29.7642, -5.5975) (-29.7745, -5.6028) (-29.7847, -5.6081) (-29.7951, -5.6134) (-29.8054, -5.6188) (-29.8158, -5.6242) (-29.8262, -5.6296) (-29.8366, -5.635) (-29.847, -5.6405) (-29.8575, -5.646) (-29.868, -5.6515) (-29.8785, -5.6571) (-29.889, -5.6627) (-29.8996, -5.6683) (-29.9102, -5.674) (-29.9208, -5.6797) (-29.9314, -5.6854) (-29.9421, -5.6912) (-29.9527, -5.697) (-29.9634, -5.7028) (-29.9742, -5.7086) (-29.9849, -5.7145) (-29.9957, -5.7204) (-30.0065, -5.7263) (-30.0173, -5.7323) (-30.0281, -5.7383) (-30.039, -5.7443) (-30.0499, -5.7504) (-30.0608, -5.7565) (-30.0717, -5.7626) (-30.0826, -5.7688) (-30.0936, -5.7749) (-30.1046, -5.7811) (-30.1156, -5.7874) (-30.1266, -5.7937) (-30.1377, -5.8) (-30.1487, -5.8063) (-30.1598, -5.8127) (-30.1709, -5.8191) (-30.1821, -5.8255) (-30.1932, -5.8319) (-30.2044, -5.8384) (-30.2156, -5.8449) (-30.2268, -5.8515) (-30.238, -5.8581) (-30.2492, -5.8647) (-30.2605, -5.8713) (-30.2718, -5.878) (-30.2831, -5.8847) (-30.2944, -5.8914) (-30.3058, -5.8982) (-30.3171, -5.905) (-30.3285, -5.9118) (-30.3399, -5.9187) (-30.3513, -5.9255) (-30.3628, -5.9325) (-30.3742, -5.9394) (-30.3857, -5.9464) (-30.3972, -5.9534) (-30.4064, -5.959) (-30.4133, -5.9633) (-30.4179, -5.9661) (-30.4202, -5.9675) knots 0 0 0 0 0 0 0.00416667 0.00833333 0.0125 0.01666667 0.02083333 0.025 0.02916667 0.03333333 0.0375 0.04166667 0.04583333 0.05 0.05416667 0.05833333 0.0625 0.06666667 0.07083333 0.075 0.07916667 0.08333333 0.0875 0.09166667 0.09583333 0.1 0.10416667 0.10833333 0.1125 0.11666667 0.12083333 0.125 0.12916667 0.13333333 0.1375 0.14166667 0.14583333 0.15 0.15416667 0.15833333 0.1625 0.16666667 0.17083333 0.175 0.17916667 0.18333333 0.1875 0.19166667 0.19583333 0.2 0.20416667 0.20833333 0.2125 0.21666667 0.22083333 0.225 0.22916667 0.23333333 0.2375 0.24166667 0.24583333 0.25 0.25416667 0.25833333 0.2625 0.26666667 0.27083333 0.275 0.27916667 0.28333333 0.2875 0.29166667 0.29583333 0.3 0.30416667 0.30833333 0.3125 0.31666667 0.32083333 0.325 0.32916667 0.33333333 0.3375 0.34166667 0.34583333 0.35 0.35416667 0.35833333 0.3625 0.36666667 0.37083333 0.375 0.37916667 0.38333333 0.3875 0.39166667 0.39583333 0.4 0.40416667 0.40833333 0.4125 0.41666667 0.42083333 0.425 0.42916667 0.43333333 0.4375 0.44166667 0.44583333 0.45 0.45416667 0.45833333 0.4625 0.46666667 0.47083333 0.475 0.47916667 0.48333333 0.4875 0.49166667 0.49583333 0.5 0.50416667 0.50833333 0.5125 0.51666667 0.52083333 0.525 0.52916667 0.53333333 0.5375 0.54166667 0.54583333 0.55 0.55416667 0.55833333 0.5625 0.56666667 0.57083333 0.575 0.57916667 0.58333333 0.5875 0.59166667 0.59583333 0.6 0.60416667 0.60833333 0.6125 0.61666667 0.62083333 0.625 0.62916667 0.63333333 0.6375 0.64166667 0.64583333 0.65 0.65416667 0.65833333 0.6625 0.66666667 0.67083333 0.675 0.67916667 0.68333333 0.6875 0.69166667 0.69583333 0.7 0.70416667 0.70833333 0.7125 0.71666667 0.72083333 0.725 0.72916667 0.73333333 0.7375 0.74166667 0.74583333 0.75 0.75416667 0.75833333 0.7625 0.76666667 0.77083333 0.775 0.77916667 0.78333333 0.7875 0.79166667 0.79583333 0.8 0.80416667 0.80833333 0.8125 0.81666667 0.82083333 0.825 0.82916667 0.83333333 0.8375 0.84166667 0.84583333 0.85 0.85416667 0.85833333 0.8625 0.86666667 0.87083333 0.875 0.87916667 0.88333333 0.8875 0.89166667 0.89583333 0.9 0.90416667 0.90833333 0.9125 0.91666667 0.92083333 0.925 0.92916667 0.93333333 0.9375 0.94166667 0.94583333 0.95 0.95416667 0.95833333 0.9625 0.96666667 0.97083333 0.975 0.97916667 0.98333333 0.9875 0.99166667 0.99583333 1 1 1 1 1 1
  spline S53 degree 5 poles (28.5147, -12.1618) (28.5128, -12.16) (28.5089, -12.1562) (28.503, -12.1506) (28.4951, -12.1432) (28.4854, -12.134) (28.4756, -12.1248) (28.4658, -12.1156) (28.4561, -12.1065) (28.4464, -12.0973) (28.4366, -12.0883) (28.4269, -12.0792) (28.4172, -12.0702) (28.4075, -12.0613) (28.3978, -12.0523) (28.3882, -12.0434) (28.3785, -12.0345) (28.3689, -12.0257) (28.3593, -12.0169) (28.3496, -12.0081) (28.34, -11.9994) (28.3305, -11.9907) (28.3209, -11.982) (28.3113, -11.9734) (28.3018, -11.9648) (28.2922, -11.9562) (28.2827, -11.9477) (28.2732, -11.9392) (28.2637, -11.9307) (28.2542, -11.9223) (28.2447, -11.9139) (28.2353, -11.9055) (28.2259, -11.8972) (28.2164, -11.8889) (28.207, -11.8807) (28.1976, -11.8724) (28.1882, -11.8643) (28.1789, -11.8561) (28.1695, -11.848) (28.1602, -11.8399) (28.1509, -11.8318) (28.1416, -11.8238) (28.1323, -11.8158) (28.123, -11.8079) (28.1137, -11.8) (28.1045, -11.7921) (28.0953, -11.7843) (28.0861, -11.7765) (28.0769, -11.7687) (28.0677, -11.7609) (28.0585, -11.7532) (28.0494, -11.7456) (28.0403, -11.7379) (28.0312, -11.7303) (28.0221, -11.7228) (28.013, -11.7153) (28.0039, -11.7078) (27.9949, -11.7003) (27.9859, -11.6929) (27.9769, -11.6855) (27.9679, -11.6781) (27.9589, -11.6708) (27.95, -11.6635) (27.9411, -11.6563) (27.9322, -11.6491) (27.9233, -11.6419) (27.9144, -11.6348) (27.9055, -11.6276) (27.8967, -11.6206) (27.8879, -11.6135) (27.8791, -11.6065) (27.8704, -11.5996) (27.8616, -11.5927) (27.8529, -11.5858) (27.8442, -11.5789) (27.8355, -11.5721) (27.8268, -11.5653) (27.8182, -11.5585) (27.8096, -11.5518) (27.801, -11.5452) (27.7924, -11.5385) (27.7838, -11.5319) (27.7753, -11.5253) (27.7668, -11.5188) (27.7583, -11.5123) (27.7498, -11.5058) (27.7414, -11.4994) (27.733, -11.493) (27.7246, -11.4867) (27.7162, -11.4803) (27.7078, -11.4741) (27.6995, -11.4678) (27.6912, -11.4616) (27.6829, -11.4554) (27.6747, -11.4493) (27.6665, -11.4432) (27.6582, -11.4371) (27.6501, -11.4311) (27.6419, -11.4251) (27.6338, -11.4192) (27.6257, -11.4132) (27.6176, -11.4074) (27.6096, -11.4015) (27.6015, -11.3957) (27.5936, -11.3899) (27.5856, -11.3842) (27.5776, -11.3785) (27.5697, -11.3728) (27.5618, -11.3672) (27.554, -11.3616) (27.5462, -11.3561) (27.5384, -11.3506) (27.5306, -11.3451) (27.5228, -11.3396) (27.5151, -11.3342) (27.5074, -11.3289) (27.4998, -11.3235) (27.4922, -11.3183) (27.4846, -11.313) (27.477, -11.3078) (27.4695, -11.3026) (27.462, -11.2975) (27.4545, -11.2924) (27.447, -11.2873) (27.4396, -11.2823) (27.4323, -11.2773) (27.4249, -11.2723) (27.4176, -11.2674) (27.4103, -11.2625) (27.4031, -11.2577) (27.3958, -11.2529) (27.3887, -11.2481) (27.3815, -11.2434) (27.3744, -11.2387) (27.3673, -11.234) (27.3603, -11.2294) (27.3533, -11.2248) (27.3463, -11.2203) (27.3393, -11.2158) (27.3324, -11.2113) (27.3256, -11.2069) (27.3187, -11.2025) (27.3119, -11.1982) (27.3052, -11.1939) (27.2985, -11.1896) (27.2918, -11.1854) (27.2851, -11.1812) (27.2785, -11.177) (27.272, -11.1729) (27.2654, -11.1688) (27.259, -11.1648) (27.2525, -11.1608) (27.2461, -11.1568) (27.2397, -11.1529) (27.2334, -11.149) (27.2271, -11.1451) (27.2209, -11.1413) (27.2147, -11.1376) (27.2085, -11.1338) (27.2024, -11.1301) (27.1963, -11.1265) (27.1903, -11.1229) (27.1843, -11.1193) (27.1784, -11.1158) (27.1725, -11.1123) (27.1666, -11.1088) (27.1608, -11.1054) (27.155, -11.102) (27.1493, -11.0987) (27.1436, -11.0954) (27.138, -11.0921) (27.1324, -11.0889) (27.1269, -11.0857) (27.1214, -11.0826) (27.116, -11.0795) (27.1106, -11.0764) (27.1053, -11.0734) (27.1, -11.0704) (27.0948, -11.0675) (27.0896, -11.0646) (27.0845, -11.0617) (27.0794, -11.0589) (27.0744, -11.0561) (27.0694, -11.0534) (27.0645, -11.0507) (27.0597, -11.048) (27.0549, -11.0454) (27.0501, -11.0428) (27.0454, -11.0403) (27.0408, -11.0378) (27.0362, -11.0353) (27.0317, -11.0329) (27.0272, -11.0306) (27.0228, -11.0282) (27.0185, -11.0259) (27.0142, -11.0237) (27.01, -11.0215) (27.0058, -11.0193) (27.0017, -11.0172) (26.9977, -11.0151) (26.9937, -11.0131) (26.9898, -11.0111) (26.986, -11.0091) (26.9822, -11.0072) (26.9785, -11.0053) (26.9748, -11.0035) (26.9713, -11.0017) (26.9678, -10.9999) (26.9643, -10.9982) (26.961, -10.9966) (26.9577, -10.9949) (26.9544, -10.9934) (26.9513, -10.9918) (26.9482, -10.9903) (26.9452, -10.9889) (26.9423, -10.9875) (26.9394, -10.9861) (26.9366, -10.9848) (26.9339, -10.9835) (26.9313, -10.9823) (26.9288, -10.9811) (26.9263, -10.9799) (26.924, -10.9788) (26.9217, -10.9778) (26.9195, -10.9768) (26.9173, -10.9758) (26.9153, -10.9749) (26.9134, -10.974) (26.9115, -10.9731) (26.9097, -10.9724) (26.908, -10.9716) (26.9065, -10.9709) (26.905, -10.9702) (26.9036, -10.9696) (26.9023, -10.9691) (26.9011, -10.9685) (26.9, -10.9681) (26.899, -10.9676) (26.8981, -10.9672) (26.8973, -10.9669) (26.8966, -10.9666) (26.8961, -10.9664) (26.8958, -10.9663) (26.8956, -10.9662) (26.8955, -10.9662) knots -1 -1 -1 -1 -1 -1 -0.99583333 -0.99166667 -0.9875 -0.98333333 -0.97916667 -0.975 -0.97083333 -0.96666667 -0.9625 -0.95833333 -0.95416667 -0.95 -0.94583333 -0.94166667 -0.9375 -0.93333333 -0.92916667 -0.925 -0.92083333 -0.91666667 -0.9125 -0.90833333 -0.90416667 -0.9 -0.89583333 -0.89166667 -0.8875 -0.88333333 -0.87916667 -0.875 -0.87083333 -0.86666667 -0.8625 -0.85833333 -0.85416667 -0.85 -0.84583333 -0.84166667 -0.8375 -0.83333333 -0.82916667 -0.825 -0.82083333 -0.81666667 -0.8125 -0.80833333 -0.80416667 -0.8 -0.79583333 -0.79166667 -0.7875 -0.78333333 -0.77916667 -0.775 -0.77083333 -0.76666667 -0.7625 -0.75833333 -0.75416667 -0.75 -0.74583333 -0.74166667 -0.7375 -0.73333333 -0.72916667 -0.725 -0.72083333 -0.71666667 -0.7125 -0.70833333 -0.70416667 -0.7 -0.69583333 -0.69166667 -0.6875 -0.68333333 -0.67916667 -0.675 -0.67083333 -0.66666667 -0.6625 -0.65833333 -0.65416667 -0.65 -0.64583333 -0.64166667 -0.6375 -0.63333333 -0.62916667 -0.625 -0.62083333 -0.61666667 -0.6125 -0.60833333 -0.60416667 -0.6 -0.59583333 -0.59166667 -0.5875 -0.58333333 -0.57916667 -0.575 -0.57083333 -0.56666667 -0.5625 -0.55833333 -0.55416667 -0.55 -0.54583333 -0.54166667 -0.5375 -0.53333333 -0.52916667 -0.525 -0.52083333 -0.51666667 -0.5125 -0.50833333 -0.50416667 -0.5 -0.49583333 -0.49166667 -0.4875 -0.48333333 -0.47916667 -0.475 -0.47083333 -0.46666667 -0.4625 -0.45833333 -0.45416667 -0.45 -0.44583333 -0.44166667 -0.4375 -0.43333333 -0.42916667 -0.425 -0.42083333 -0.41666667 -0.4125 -0.40833333 -0.40416667 -0.4 -0.39583333 -0.39166667 -0.3875 -0.38333333 -0.37916667 -0.375 -0.37083333 -0.36666667 -0.3625 -0.35833333 -0.35416667 -0.35 -0.34583333 -0.34166667 -0.3375 -0.33333333 -0.32916667 -0.325 -0.32083333 -0.31666667 -0.3125 -0.30833333 -0.30416667 -0.3 -0.29583333 -0.29166667 -0.2875 -0.28333333 -0.27916667 -0.275 -0.27083333 -0.26666667 -0.2625 -0.25833333 -0.25416667 -0.25 -0.24583333 -0.24166667 -0.2375 -0.23333333 -0.22916667 -0.225 -0.22083333 -0.21666667 -0.2125 -0.20833333 -0.20416667 -0.2 -0.19583333 -0.19166667 -0.1875 -0.18333333 -0.17916667 -0.175 -0.17083333 -0.16666667 -0.1625 -0.15833333 -0.15416667 -0.15 -0.14583333 -0.14166667 -0.1375 -0.13333333 -0.12916667 -0.125 -0.12083333 -0.11666667 -0.1125 -0.10833333 -0.10416667 -0.1 -0.09583333 -0.09166667 -0.0875 -0.08333333 -0.07916667 -0.075 -0.07083333 -0.06666667 -0.0625 -0.05833333 -0.05416667 -0.05 -0.04583333 -0.04166667 -0.0375 -0.03333333 -0.02916667 -0.025 -0.02083333 -0.01666667 -0.0125 -0.00833333 -0.00416667 0 0 0 0 0 0